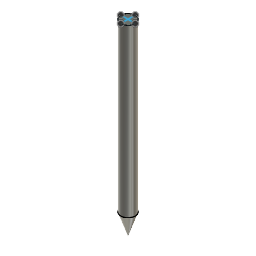
PenPlotter (Autodesk Fusion 360 archive; units mm, degrees)
design "Pen"
part number: 2026-07-09-13-50-47-869
Autodesk Fusion 360 part; units mm, degrees
sketch "Sketch1" plane through (0, 0, 0) normal (0, 0, 1) x (1, 0, 0)
  circle A0 centre (0, 0) radius 4.75
  dimension "d1" = 9.5
  constraint coincident A0.centre origin
  measures "d1" diameter of A0
extrude "Extrude1" add sketch "Sketch1" along normal blind 109
sketch "Sketch2" plane through (0, 0, 0) normal (0, 1, 0) x (1, 0, 0)
  line L0 (-4.75, -109) -> (0, -123)
  line L1 (-4.75, -109) -> (0, -109)
  line L2 (0, -109) -> (0, -123)
  constraint horizontal L1
  constraint perpendicular L1 L2
revolve "Revolve1" add sketch "Sketch2" angle 360 about axis through (0, 0, 0) along (0, 0, -1)
move_body "Move1" bodies 1 to x (-1, 0, 0) y (0, 1, 0) z (0, 0, -1) at (0, 0, 109)
sketch "Sketch3" plane through (0, 0, 109) normal (0, 0, 1) x (-1, 0, 0)
  circle A0 centre (0, 0) radius 4.75
  line L0 (0, -4.75) -> (0, 4.75)
  line L1 (-4.75, 0) -> (4.75, 0)
  constraint coincident A0 L0.start
  constraint coincident A0 L0.end
  constraint vertical L0
  constraint coincident A0 L1.start
  constraint coincident A0 L1.end
  constraint perpendicular L0 L1
